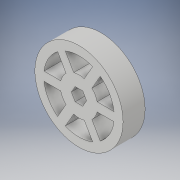
# Autodesk Inventor part: RobotArm Wheel2
Saved by Autodesk Inventor 2018 (Build 220112000, 112)
## iProperties
Created: 2018-01-13
Part Number: RobotArm Wheel2
Material: Generic
Document SubType Name: Modeling
Designer: lopez.xavier
Density: 1 g/cm^3
Appearance: Default
Author: lopez.xavier
Autodesk Inventor part; units mm, degrees
ref_plane "YZ Plane" through (0, 0, 0) normal (1, 0, 0) x (0, 1, 0)
ref_plane "XZ Plane" through (0, 0, 0) normal (0, 1, 0) x (-1, 0, 0)
ref_plane "XY Plane" through (0, 0, 0) normal (0, 0, 1) x (1, 0, 0)
sketch "Sketch1" plane through (0, 0, 0) normal (0, 0, 1) x (1, 0, 0)
  line L0 (2.1997, 3.81) -> (4.3994, 0)
  line L1 (4.3994, 0) -> (2.1997, -3.81)
  line L2 (2.1997, -3.81) -> (-2.1997, -3.81)
  line L3 (-2.1997, -3.81) -> (-4.3994, 0)
  line L4 (-4.3994, 0) -> (-2.1997, 3.81)
  line L5 (-2.1997, 3.81) -> (2.1997, 3.81)
  line L6 (0, 0) -> (1.743, 0)
  circle A0 centre (0, 0) radius 10.795
  circle A1 centre (0, 0) radius 25.4
  circle A2 centre (0, 0) radius 20.32
  line L7 (-4.3994, 0) -> (-20.32, 0)
  line L8 (-2.1997, 3.81) -> (-10.16, 17.5976)
  line L9 (2.1997, 3.81) -> (10.16, 17.5976)
  line L10 (4.3994, 0) -> (20.32, 0)
  line L11 (2.1997, -3.81) -> (10.16, -17.5976)
  line L12 (-2.1997, -3.81) -> (-10.16, -17.5976)
  line L13 (-2.9329, 2.54) -> (-20.1606, 2.54)
  line L14 (-2.9329, -2.54) -> (-20.1606, -2.54)
  line L15 (-3.6662, -1.27) -> (-12.28, -16.1896)
  line L16 (0.7332, -3.81) -> (-7.8806, -18.7296)
  line L17 (-0.7332, -3.81) -> (7.8806, -18.7296)
  line L18 (3.6662, -1.27) -> (12.28, -16.1896)
  line L19 (2.9329, 2.54) -> (20.1606, 2.54)
  line L20 (2.9329, -2.54) -> (20.1606, -2.54)
  line L21 (-7.4457, 7.8163) -> (-12.28, 16.1896)
  line L22 (-3.0463, 10.3563) -> (-7.8806, 18.7296)
  line L23 (-0.7332, 3.81) -> (7.8806, 18.7296)
  line L24 (3.6662, 1.27) -> (12.28, 16.1896)
  dimension "d0" = 7.62
  dimension "d1" = 21.59
  dimension "d2" = 50.8
  dimension "d3" = 5.08
  dimension "d4" = 120
  dimension "d5" = 120
  dimension "d6" = 120
  dimension "d7" = 120
  dimension "d8" = 5.08
  dimension "d9" = 2.54
  dimension "d10" = 5.08
  dimension "d11" = 2.54
  dimension "d13" = 2.54
  dimension "d14" = 5.08
  dimension "d15" = 5.08
  dimension "d17" = 2.54
  dimension "d18" = 2.54
  dimension "d19" = 2.54
  dimension "d20" = 5.08
  dimension "d21" = 2.54
  constraints: 50 end point, 13 parallel, 10 point on line, 4 coincident, 3 horizontal, 2 centre point, 2 point on circle, 33 other
  measures "d0" distance between parallel lines of L2 L5
  measures "d1" diameter of A0
  measures "d2" diameter of A1
  measures "d4" angle of L8 L5
  measures "d5" angle of L3 L12
  measures "d6" angle of L1 L11
  measures "d7" angle of L0 L9
  measures "d8" distance between parallel lines of L13 L14
  measures "d9" distance between parallel lines of L7 L14
  measures "d10" distance between parallel lines of L15 L16
  measures "d11" distance between parallel lines of L15 L12
  measures "d13" distance between parallel lines of L17 L11
  measures "d14" distance between parallel lines of L17 L18
  measures "d15" distance between parallel lines of L19 L20
  measures "d17" distance between parallel lines of L10 L20
  measures "d18" distance between parallel lines of L8 L22
  measures "d19" distance between parallel lines of L8 L21
  measures "d20" distance between parallel lines of L24 L23
  measures "d21" distance between parallel lines of L9 L23
extrude "Extrusion1" add sketch "Sketch1" along normal blind 12.7 contours L9 A0 L24 L19 L0 | L5 L23 A0 L9 | L19 L24 L0 | L5 L8 A0 L23 | L9 A2 L24 A0 | A0 L23 A2 L9 | L24 L19 A0 L10 L0 | L24 A0 L19 | L4 L13 A0 L8 | L10 A0 L20 L18 L1 | L19 A2 L10 A0 | L4 L7 A0 L13 | L8 A2 L22 A0 | A0 L21 A2 L8 | L18 L20 L1 | L10 A2 L20 A0 | L3 L15 L14 A0 L7 | A0 L7 A2 L13 | L20 L18 A0 L11 L1 | L20 A0 L18 | L3 L14 L15 | A0 L14 A2 L7 | L11 A0 L17 L16 L2 | L18 A2 L11 A0 | L3 L12 A0 L15 L14 | L15 A0 L14 | L16 L17 L2 | L11 A2 L17 A0 | L2 L17 L16 A0 L12 | A0 L12 A2 L15 | L17 A0 L16 | A0 L16 A2 L12 | A1
equation "\"d5\" = d4"
equation "\"d6\" = d4"
equation "\"d7\" = d4"
body "Solid1"
